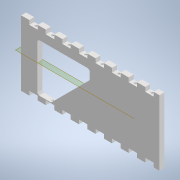
# Autodesk Inventor part: 00_Baseplate_Simmo_side2
Saved by Autodesk Inventor 2022 (Build 260153000, 153)
## iProperties
Created: 2022-05-05
Part Number: 00_Baseplate_Simmo_side2
Material: Generic
Document SubType Name: Modeling
Designer: wanghaoran
Density: 1 g/cm^3
Appearance: Default
Author: wanghaoran
Autodesk Inventor part; units mm, degrees
ref_plane "YZ Plane" through (0, 0, 0) normal (1, 0, 0) x (0, 1, 0)
ref_plane "XZ Plane" through (0, 0, 0) normal (0, 1, 0) x (-1, 0, 0)
ref_plane "XY Plane" through (0, 0, 0) normal (0, 0, 1) x (1, 0, 0)
sketch "Sketch1" plane through (0, 0, 0) normal (0, 0, 1) x (1, 0, 0)
  line L0 (0, -120) -> (0, 155.2673) projected
  line L1 (-130, 0) -> (-130, 5) projected
  line L2 (-10, 5) -> (0, 5) projected
  line L3 (0, -74) -> (-9.8, -74) projected
  line L4 (-130, 5) -> (-120, 5) projected
  line L5 (-120.2, -74) -> (-129.8, -74) projected
  line L6 (-129.8, -69) -> (-129.8, -74) projected
  line L7 (0, 5) -> (-170.1, 5)
  line L8 (-170.1, 5) -> (-170.1, -74)
  line L9 (-170.1, -74) -> (0, -74)
  line L10 (0, -74) -> (0, 5)
  line L11 (-155.5538, -1) -> (-155.5538, 5) projected
  line L12 (-170.1, 0) -> (-170.1, 5) projected
  point P0 (0, 0)
  dimension "d27" = 0
  constraints: 8 end point, 2 parallel, 1 horizontal, 1 perpendicular
  measures "d27" distance between parallel lines of L12 L8
extrude "Extrusion1" add sketch "Sketch1" along normal blind 6
sketch "Sketch2" plane through (0, 0, 6) normal (0, 0, 1) x (1, 0, 0)
  line L0 (-10, 0) -> (-10, 5) projected
  line L1 (0, 5) -> (-170.1, 5) projected
  line L2 (-20, 0) -> (-10, 0) projected
  line L3 (-20, 5) -> (-20, 0) projected
  line L4 (-9.9, 5) -> (-9.9, 0)
  line L5 (-20.1, 0) -> (-20.1, 5)
  line L6 (-10, 0) -> (-9.9, 0)
  line L7 (-20, 0) -> (-20.1, 0)
  point P0 (-130, 5)
  constraints: 8 end point, 1 perpendicular, 1 point on line
extrude "Extrusion2" cut sketch "Sketch2" against normal blind 6
sketch "Sketch3" plane through (-20.1, 0, 6) normal (0, 1, 0) x (1, 0, 0)
  circle A0 centre (5.1, 3) radius 1.5 projected
  point P0 (20.1, 6)
hole "Hole1" at (-15, 0, 3) direction (0, -1, 0) diameter 2.8 depth 20
pattern_linear "Rectangular Pattern2" count 9 spacing 20 along (-1, 0, 0) of "Extrusion2", "Hole1"
ref_plane "Work Plane1" through (-170.1, -34.5, 0) normal (0, -1, 0) x (1, 0, 0)
mirror "Mirror1" about plane through (-170.1, -34.5, 0) normal (0, -1, 0) of "Extrusion2", "Hole1", "Rectangular Pattern2"
sketch "Skizze4" plane through (0, 0, 6) normal (0, 0, 1) x (1, 0, 0)
  line L0 (-2.3877, 5) -> (-2.3877, -75) projected
  line L1 (16.4895, -81.7963) -> (-2.8877, -81.7963)
  line L2 (-2.8877, -81.7963) -> (-2.8877, 13.3495)
  line L3 (-2.8877, 13.3495) -> (16.4895, 13.3495)
  line L4 (16.4895, 13.3495) -> (16.4895, -81.7963)
  point P0 (0, 0)
  dimension "d23" = 0.5
  constraints: 8 end point, 2 parallel, 1 horizontal, 1 perpendicular
  measures "d23" distance between parallel lines of L0 L2
extrude "Extrusion3" cut sketch "Skizze4" against normal blind 10
sketch "Skizze5" plane through (0, 0, 6) normal (0, 0, 1) x (1, 0, 0)
  ellipse E0 centre (-101.986, -20.3375) end of major axis (-101.986, -27.7035) minor radius 7.2541 projected
  ellipse E1 centre (-140.4361, -58.0565) end of major axis (-140.4361, -65.4225) minor radius 7.2541 projected
  line L0 (-150.4361, -68.0565) -> (-91.986, -68.0565)
  line L1 (-86.986, -21.3155) -> (-86.986, -5)
  line L2 (-86.986, -5) -> (-150.4361, -5)
  line L3 (-150.4361, -5) -> (-150.4361, -68.0565)
  line L4 (-133.727, -68.0565) -> (-86.986, -21.3155)
  line L5 (-133.727, -68.0565) -> (-67.6252, -68.0565) construction
  line L6 (-86.986, -5) -> (-150.4361, -5)
  line L7 (-150.4361, -5) -> (-150.4361, -10)
  line L8 (-150.4361, -10) -> (-86.986, -10)
  line L9 (-86.986, -10) -> (-86.986, -5)
  point P0 (0, 0)
  dimension "d28" = 15
  dimension "d29" = 10
  dimension "d30" = 10
  dimension "d33" = 45
  dimension "d34" = 5
  constraints: 20 end point, 4 parallel, 3 horizontal, 2 perpendicular, 2 point on line, 1 equal length, 2 other
  measures "d28" distance from line of L1 point (-101.986, -20.337)
  measures "d29" distance from line of L3 point (-140.436, -58.056)
  measures "d30" distance from line of L0 point (-140.436, -58.056)
  measures "d33" angle of L5 L4
  measures "d34" distance of L7.end L6.end
extrude "Extrusion4" cut sketch "Skizze5" against normal blind 10 contours E0 | E1 | L3 L8 L1 L4 L0
fillet "Rundung1" radius 3 4 edges at (-86.986, -10, 3) (-86.986, -21.3155, 3) (-150.4361, -68.0565, 3) (-150.4361, -10, 3)
body "Solid1"
